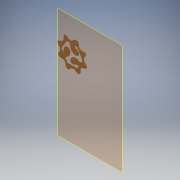
# Autodesk Inventor part: logoDraw
Saved by Autodesk Inventor 2019 (Build 230136000, 136)
## iProperties
Created: 2019-01-25
Part Number: logoDraw
Material: Wood (Cherry)
Document SubType Name: Modeling
Designer: gaincarlo
Density: 0.63 g/cm^3
Appearance: Cherry - Natural Low Gloss
Author: gaincarlo
Autodesk Inventor part; units mm, degrees
ref_plane "YZ Plane" through (0, 0, 0) normal (1, 0, 0) x (0, 1, 0)
ref_plane "XZ Plane" through (0, 0, 0) normal (0, 1, 0) x (-1, 0, 0)
ref_plane "XY Plane" through (0, 0, 0) normal (0, 0, 1) x (1, 0, 0)
ref_plane "Work Plane1" through (0, 0, 0) normal (0, 0, 1) x (1, 0, 0)
sketch "Sketch1" plane through (0, 0, 0) normal (0, 0, 1) x (1, 0, 0)
  line L0 (-320.6659, 365.07) -> (-303.6236, 365.07) projected
  spline S0 degree 3 poles (-320.9918, 365.6066) (-321.0765, 365.7292) (-320.8908, 365.3877) (-320.6659, 365.07) knots 2.320993 2.320993 2.320993 2.320993 3 3 3 3 projected
  spline S1 degree 3 poles (-352.5793, 368.487) (-340.4491, 375.5323) (-326.8416, 374.8317) (-320.9918, 365.6066) knots 3 3 3 3 3.981304 3.981304 3.981304 3.981304 projected
  spline S2 degree 3 poles (-366.293, 340.5724) (-371.0762, 348.8109) (-364.9349, 361.3096) (-352.5793, 368.487) knots 4 4 4 4 5 5 5 5 projected
  spline S3 degree 3 poles (-335.2478, 338.6495) (-347.6077, 331.4693) (-361.5095, 332.3307) (-366.293, 340.5724) knots 5 5 5 5 6 6 6 6 projected
  line L1 (-330.2832, 342.0297) -> (-335.2478, 338.6495) projected
  line L2 (-316.9989, 342.0297) -> (-330.2832, 342.0297) projected
  line L3 (-327.0734, 324.5796) -> (-316.9989, 342.0297) projected
  line L4 (-389.8551, 324.5796) -> (-327.0734, 324.5796) projected
  line L5 (-391.6641, 325.7587) -> (-389.8551, 324.5796) projected
  line L6 (-399.6179, 339.5077) -> (-391.6641, 325.7587) projected
  line L7 (-391.0968, 354.2667) -> (-399.6179, 339.5077) projected
  spline S4 degree 3 poles (-390.4692, 354.2806) (-390.3206, 354.2927) (-390.7092, 354.3026) (-391.0968, 354.2667) knots 2.320993 2.320993 2.320993 2.320993 3 3 3 3 projected
  spline S5 degree 3 poles (-372.1809, 380.196) (-372.1446, 366.1683) (-379.5551, 354.7342) (-390.4692, 354.2806) knots 3 3 3 3 3.981304 3.981304 3.981304 3.981304 projected
  spline S6 degree 3 poles (-389.4988, 406.0297) (-379.9724, 406.0529) (-372.2189, 394.485) (-372.1809, 380.196) knots 4 4 4 4 5 5 5 5 projected
  spline S7 degree 3 poles (-406.6867, 380.1052) (-406.725, 394.3993) (-399.028, 406.008) (-389.4988, 406.0297) knots 5 5 5 5 6 6 6 6 projected
  line L8 (-406.2417, 374.1157) -> (-406.6867, 380.1052) projected
  line L9 (-412.8838, 362.6111) -> (-406.2417, 374.1157) projected
  line L10 (-422.9588, 380.0609) -> (-412.8838, 362.6111) projected
  line L11 (-391.568, 434.4315) -> (-422.9588, 380.0609) projected
  line L12 (-389.6423, 435.4086) -> (-391.568, 434.4315) projected
  line L13 (-373.7584, 435.4223) -> (-389.6423, 435.4086) projected
  line L14 (-365.2373, 420.6633) -> (-373.7584, 435.4223) projected
  spline S8 degree 3 poles (-365.5391, 420.1128) (-365.6029, 419.9781) (-365.4, 420.3097) (-365.2373, 420.6633) knots 2.320993 2.320993 2.320993 2.320993 3 3 3 3 projected
  spline S9 degree 3 poles (-352.2398, 391.317) (-364.4063, 398.2994) (-370.6033, 410.4341) (-365.5391, 420.1128) knots 3 3 3 3 3.981304 3.981304 3.981304 3.981304 projected
  spline S10 degree 3 poles (-321.2082, 393.3979) (-325.9513, 385.1362) (-339.8462, 384.2054) (-352.2398, 391.317) knots 4 4 4 4 5 5 5 5 projected
  spline S11 degree 3 poles (-335.0655, 421.2453) (-322.6673, 414.1314) (-316.4624, 401.6613) (-321.2082, 393.3979) knots 5 5 5 5 6 6 6 6 projected
  line L15 (-340.4751, 423.8546) -> (-335.0655, 421.2453) projected
  line L16 (-347.1173, 435.3592) -> (-340.4751, 423.8546) projected
  line L17 (-326.9678, 435.3595) -> (-347.1173, 435.3592) projected
  line L18 (-295.577, 380.9889) -> (-326.9678, 435.3595) projected
  line L19 (-295.6936, 378.8327) -> (-295.577, 380.9889) projected
  line L20 (-303.6236, 365.07) -> (-295.6936, 378.8327) projected
  line L21 (-427.984, 366.6864) -> (-429.2569, 380) projected
  line L22 (-441.4092, 343.8238) -> (-427.984, 366.6864) projected
  line L23 (-435.1382, 332.0107) -> (-441.4092, 343.8238) projected
  line L24 (-408.6792, 330.3208) -> (-435.1382, 332.0107) projected
  line L25 (-398.3649, 321.8068) -> (-408.6792, 330.3208) projected
  line L26 (-391.6916, 296.1474) -> (-398.3649, 321.8068) projected
  line L27 (-378.9043, 292.2286) -> (-391.6916, 296.1474) projected
  line L28 (-359, 309.7431) -> (-378.9043, 292.2286) projected
  line L29 (-345.6864, 311.016) -> (-359, 309.7431) projected
  line L30 (-322.8238, 297.5908) -> (-345.6864, 311.016) projected
  line L31 (-311.0107, 303.8618) -> (-322.8238, 297.5908) projected
  line L32 (-309.3208, 330.3208) -> (-311.0107, 303.8618) projected
  line L33 (-300.8068, 340.6351) -> (-309.3208, 330.3208) projected
  line L34 (-275.1474, 347.3084) -> (-300.8068, 340.6351) projected
  line L35 (-271.2286, 360.0957) -> (-275.1474, 347.3084) projected
  line L36 (-288.7431, 380) -> (-271.2286, 360.0957) projected
  line L37 (-290.016, 393.3136) -> (-288.7431, 380) projected
  line L38 (-276.5908, 416.1762) -> (-290.016, 393.3136) projected
  line L39 (-282.8618, 427.9893) -> (-276.5908, 416.1762) projected
  line L40 (-309.3208, 429.6792) -> (-282.8618, 427.9893) projected
  line L41 (-319.6351, 438.1932) -> (-309.3208, 429.6792) projected
  line L42 (-326.3084, 463.8526) -> (-319.6351, 438.1932) projected
  line L43 (-339.0957, 467.7714) -> (-326.3084, 463.8526) projected
  line L44 (-359, 450.2569) -> (-339.0957, 467.7714) projected
  line L45 (-372.3136, 448.984) -> (-359, 450.2569) projected
  line L46 (-395.1762, 462.4092) -> (-372.3136, 448.984) projected
  line L47 (-406.9893, 456.1382) -> (-395.1762, 462.4092) projected
  line L48 (-408.6792, 429.6792) -> (-406.9893, 456.1382) projected
  line L49 (-417.1932, 419.3649) -> (-408.6792, 429.6792) projected
  line L50 (-442.8526, 412.6916) -> (-417.1932, 419.3649) projected
  line L51 (-446.7714, 399.9043) -> (-442.8526, 412.6916) projected
  line L52 (-429.2569, 380) -> (-446.7714, 399.9043) projected
  point P0 (0, 0)
extrude "Extrusion1" add sketch "Sketch1" against normal blind 4
body "Solid1"
